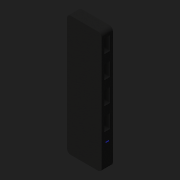
# Autodesk Inventor part: USB Hub
Saved by Autodesk Inventor 2017 SP1 (Build 210196100, 196)
## iProperties
Created: 2017-09-20
Part Number: USB Hub
Material: ABS Plastic
Document SubType Name: Modeling
Designer: Zach
Density: 1.06 g/cm^3
Appearance: Black
Author: Zach
Autodesk Inventor part; units mm, degrees
ref_plane "YZ Plane" through (0, 0, 0) normal (1, 0, 0) x (0, 1, 0)
ref_plane "XZ Plane" through (0, 0, 0) normal (0, 1, 0) x (-1, 0, 0)
ref_plane "XY Plane" through (0, 0, 0) normal (0, 0, 1) x (1, 0, 0)
sketch "Sketch1" plane through (0, 0, 0) normal (0, 0, 1) x (1, 0, 0)
  line L0 (0, 0) -> (30.734, 0)
  line L1 (30.734, 0) -> (30.734, -106.934)
  line L2 (30.734, -106.934) -> (0, -106.934)
  line L3 (0, -106.934) -> (0, 0)
  dimension "d0" = 30.734
  dimension "d1" = 106.934
  constraints: 8 end point, 2 parallel, 1 horizontal, 1 perpendicular
  measures "d0" distance of L1.end L2.end
  measures "d1" distance of L0.end L1.end
extrude "Extrusion1" add sketch "Sketch1" along normal blind 10
fillet "Fillet1" radius 3.175 4 edges at (0, 0, 5) (30.734, 0, 5) (30.734, -106.934, 5) (0, -106.934, 5)
sketch "Sketch2" plane through (30.734, -103.759, 0) normal (1, 0, 0) x (0, 0, -1)
  line L0 (-7.5, 26.825) -> (-2.5, 26.825)
  line L1 (-2.5, 26.825) -> (-2.5, 38.825)
  line L2 (-2.5, 38.825) -> (-7.5, 38.825)
  line L3 (-7.5, 38.825) -> (-7.5, 26.825)
  line L4 (-10, -3.175) -> (0, -3.175) projected
  line L5 (-10, -3.175) -> (-10, 0) projected
  line L6 (-7.5, 46.825) -> (-2.5, 46.825)
  line L7 (-2.5, 46.825) -> (-2.5, 58.825)
  line L8 (-2.5, 58.825) -> (-7.5, 58.825)
  line L9 (-7.5, 58.825) -> (-7.5, 46.825)
  line L10 (-7.5, 66.825) -> (-2.5, 66.825)
  line L11 (-2.5, 66.825) -> (-2.5, 78.825)
  line L12 (-2.5, 78.825) -> (-7.5, 78.825)
  line L13 (-7.5, 78.825) -> (-7.5, 66.825)
  line L14 (-7.5, 86.825) -> (-2.5, 86.825)
  line L15 (-2.5, 86.825) -> (-2.5, 98.825)
  line L16 (-2.5, 98.825) -> (-7.5, 98.825)
  line L17 (-7.5, 98.825) -> (-7.5, 86.825)
  point P0 (0, 103.759)
  point P1 (-5, 26.825)
  point P2 (-5, -3.175)
  point P3 (-5, 46.825)
  point P4 (-5, 66.825)
  point P5 (-5, 86.825)
  dimension "d5" = 30
  dimension "d6" = 12
  dimension "d7" = 5
  dimension "d10" = 20
  constraints: 32 end point, 2 midpoint, 2 parallel, 1 horizontal, 1 perpendicular, 1 vertical, 1 vertical alignment, 27 other
  measures "d5" distance between parallel lines of L4 L0
  measures "d6" distance of L2.end L0.start
  measures "d7" distance of L0.start L0.end
  measures "d10" distance of L0.start L6.start
extrude "Extrusion2" cut sketch "Sketch2" against normal blind 10
sketch "Sketch3" plane through (30.734, -103.759, 0) normal (1, 0, 0) x (0, 0, -1)
  line L0 (-6.5, 17.825) -> (-3.5, 17.825)
  line L1 (-3.5, 17.825) -> (-3.5, 18.825)
  line L2 (-3.5, 18.825) -> (-6.5, 18.825)
  line L3 (-6.5, 18.825) -> (-6.5, 17.825)
  line L4 (-10, -3.175) -> (0, -3.175) projected
  point P0 (0, 103.759)
  point P1 (-5, 17.825)
  point P2 (-5, -3.175)
  dimension "d17" = 21
  dimension "d18" = 1
  dimension "d19" = 3
  constraints: 8 end point, 2 midpoint, 2 parallel, 1 horizontal, 1 perpendicular, 1 vertical alignment
  measures "d17" distance between parallel lines of L4 L0
  measures "d18" distance from line of L2 L0.start
  measures "d19" distance of L1.end L2.end
extrude "Extrusion3" cut sketch "Sketch3" against normal blind 0.1
sketch "Sketch4" plane through (20.734, -103.759, 0) normal (1, 0, 0) x (0, 0, -1)
  line L0 (-6.5, 27.825) -> (-5.5, 27.825)
  line L1 (-5.5, 27.825) -> (-5.5, 37.825)
  line L2 (-5.5, 37.825) -> (-6.5, 37.825)
  line L3 (-6.5, 37.825) -> (-6.5, 27.825)
  line L4 (-7.5, 26.825) -> (-7.5, 38.825) projected
  line L5 (-2.5, 26.825) -> (-7.5, 26.825) projected
  line L6 (-7.5, 38.825) -> (-2.5, 38.825) projected
  line L7 (-6.5, 47.825) -> (-5.5, 47.825)
  line L8 (-5.5, 47.825) -> (-5.5, 57.825)
  line L9 (-5.5, 57.825) -> (-6.5, 57.825)
  line L10 (-6.5, 57.825) -> (-6.5, 47.825)
  line L11 (-6.5, 67.825) -> (-5.5, 67.825)
  line L12 (-5.5, 67.825) -> (-5.5, 77.825)
  line L13 (-5.5, 77.825) -> (-6.5, 77.825)
  line L14 (-6.5, 77.825) -> (-6.5, 67.825)
  line L15 (-6.5, 87.825) -> (-5.5, 87.825)
  line L16 (-5.5, 87.825) -> (-5.5, 97.825)
  line L17 (-5.5, 97.825) -> (-6.5, 97.825)
  line L18 (-6.5, 97.825) -> (-6.5, 87.825)
  point P0 (0, 103.759)
  point P1 (-6.5, 32.825)
  point P2 (-7.5, 32.825)
  point P3 (-6.5, 52.825)
  point P4 (-6.5, 72.825)
  point P5 (-6.5, 92.825)
  dimension "d24" = 1
  dimension "d25" = 1
  dimension "d26" = 1
  dimension "d29" = 20
  constraints: 32 end point, 2 midpoint, 2 parallel, 1 horizontal, 1 horizontal alignment, 1 perpendicular, 1 vertical, 27 other
  measures "d24" distance between parallel lines of L4 L3
  measures "d25" distance between parallel lines of L5 L0
  measures "d26" distance of L1.end L2.end
  measures "d29" distance of L0.start L7.start
extrude "Extrusion4" add sketch "Sketch4" along normal blind 8
sketch "Sketch5" plane through (3.175, -106.934, 0) normal (0, -1, 0) x (1, 0, 0)
  line L0 (9.192, 9) -> (15.192, 9)
  line L1 (15.192, 9) -> (15.192, 1)
  line L2 (15.192, 1) -> (9.192, 1)
  line L3 (9.192, 1) -> (9.192, 9)
  line L4 (0, 10) -> (24.384, 10) projected
  line L5 (24.384, 0) -> (0, 0) projected
  point P0 (-3.175, 0)
  point P1 (12.192, 9)
  point P2 (12.192, 10)
  dimension "d36" = 6
  dimension "d37" = 1
  dimension "d38" = 1
  constraints: 8 end point, 2 midpoint, 2 parallel, 1 horizontal, 1 perpendicular, 1 vertical alignment
  measures "d36" distance of L1.end L2.end
  measures "d37" distance between parallel lines of L4 L0
  measures "d38" distance between parallel lines of L5 L2
extrude "Extrusion5" cut sketch "Sketch5" against normal blind 5
sketch "Sketch6" plane through (12.367, -106.934, 1) normal (0, 0, 1) x (1, 0, 0)
  line L0 (6, 0) -> (0, 0) projected
  line L1 (6, 0) -> (6, 5) projected
  line L2 (6, 5) -> (0, 5) projected
  line L3 (0, 0) -> (0, 5) projected
  line L4 (-9, 0) -> (15, 0)
  line L5 (-9, 0) -> (0, 5)
  line L6 (15.192, 0) -> (-9.192, 0) projected
  line L7 (6, 5) -> (15.192, 0)
  point P0 (-12.367, 106.934)
  point P1 (3, 0)
  dimension "d41" = 24
  constraints: 6 end point, 2 midpoint, 1 horizontal
  measures "d41" distance of L4.start L4.end
extrude "Extrusion6" cut sketch "Sketch6" along normal blind 8 contours L1 L7 L6 L4 | L4 L5 L3
body "Solid1"
